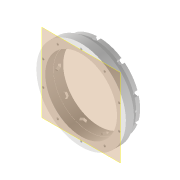
# Autodesk Inventor part: Anglerfish_3inch_tube_endpiece
Saved by Autodesk Inventor 2022 (Build 260153000, 153)
## iProperties
Created: 2022-04-12
Part Number: Anglerfish_3inch_tube_endpiece
Material: Generic
Document SubType Name: Modeling
Designer: Prakash Lab
Density: 1 g/cm^3
Appearance: Default
Author: Prakash Lab
Autodesk Inventor part; units mm, degrees
ref_plane "YZ Plane" through (0, 0, 0) normal (1, 0, 0) x (0, 1, 0)
ref_plane "XZ Plane" through (0, 0, 0) normal (0, 1, 0) x (-1, 0, 0)
ref_plane "XY Plane" through (0, 0, 0) normal (0, 0, 1) x (1, 0, 0)
ref_plane "Work Plane1" through (0, 0, -3) normal (0, 0, 1) x (0, -1, 0)
sketch "Sketch1" plane through (0, 0, -3) normal (0, 0, 1) x (0, -1, 0)
  circle A0 centre (0, 0) radius 44.3 projected
  circle A1 centre (0, 0) radius 44.6
  circle A2 centre (0, 0) radius 55.6
  point P0 (0, 0)
  dimension "d0" = 0.3
  dimension "d1" = 11
  constraints: 2 centre point
  measures "d0" radial gap between concentric circles of A0 A1
  measures "d1" radial gap between concentric circles of A1 A2
extrude "Extrusion1" add sketch "Sketch1" against normal blind 10 contours A2
sketch "Sketch2" plane through (0, 0, -13) normal (0, 0, -1) x (-1, 0, 0)
  circle A0 centre (0, 0) radius 44.3 projected
  circle A1 centre (0, 0) radius 51.3
  point P0 (0, 0)
  dimension "d4" = 7
  constraints: 1 centre point
  measures "d4" radial gap between concentric circles of A0 A1
extrude "Extrusion2" add sketch "Sketch2" along normal blind 12
sketch "Sketch3" plane through (0, 0, 0) normal (1, 0, 0) x (0, 1, 0)
  line L0 (-51.3, -25) -> (51.3, -25) projected
  line L1 (51.3, -13) -> (-51.3, -13) projected
  line L2 (-55.6, -13) -> (55.6, -13) projected
  line L3 (55.6, -3) -> (-55.6, -3) projected
  circle A0 centre (0, -19) radius 1.45
  point P0 (0, 0)
  dimension "d7" = 2.9
  dimension "d8" = 6
  constraints: 1 centre point
  measures "d7" diameter of A0
  measures "d8" distance from line of A0.centre L0
extrude "Extrusion3" cut sketch "Sketch3" along normal through all both and the other way through all
sketch "Sketch4" plane through (0, 0, 0) normal (1, 0, 0) x (0, 1, 0)
  line L0 (-1.9269, -22.2506) -> (-3.8033, -19.0006)
  line L1 (-3.8033, -19.0006) -> (-1.9269, -15.7506)
  line L2 (-1.9269, -15.7506) -> (1.8259, -15.7506)
  line L3 (1.8259, -15.7506) -> (3.7023, -19.0006)
  line L4 (3.7023, -19.0006) -> (1.8259, -22.2506)
  line L5 (1.8259, -22.2506) -> (-1.9269, -22.2506)
  line L6 (-55.6, -13) -> (55.6, -13) projected
  point P0 (0, 0)
  point P1 (-0.0505, -19.0006)
  dimension "d11" = 6.5
  constraints: 12 end point, 1 parallel, 14 other
  measures "d11" distance between parallel lines of L5 L2
extrude "Extrusion4" cut sketch "Sketch4" along normal mid plane 96
chamfer "Chamfer1" distance 4 distance2 7 1 edges at (51.3, 0, -13) measured on face at (51.8, 0, -13)
pattern_circular "Circular Pattern1" count 10 over 360 about axis through (0, 0, -13) along (0, 0, -1) of "Extrusion4"
sketch "Sketch5" plane through (0, 0, -3) normal (0, 0, 1) x (1, 0, 0)
  circle A0 centre (0, 0) radius 55.6 projected
  circle A1 centre (0, 0) radius 44.3 projected
  circle A2 centre (0, 0) radius 49.6 construction
  circle A3 centre (0, 49.6) radius 1.45
  point P0 (0, 0)
  dimension "d20" = 6
  dimension "d21" = 2.9
  constraints: 1 centre point, 1 vertical alignment, 2 other
  measures "d21" diameter of A3
extrude "Extrusion5" cut sketch "Sketch5" against normal blind 96 contours A3
sketch "Sketch6" plane through (0, 0, -25) normal (0, 0, -1) x (-1, 0, 0)
  circle A0 centre (0, 49.6) radius 1.45 projected
  line L0 (1.7321, 52.6) -> (3.4641, 49.6)
  line L1 (3.4641, 49.6) -> (1.7321, 46.6)
  line L2 (1.7321, 46.6) -> (-1.7321, 46.6)
  line L3 (-1.7321, 46.6) -> (-3.4641, 49.6)
  line L4 (-3.4641, 49.6) -> (-1.7321, 52.6)
  line L5 (-1.7321, 52.6) -> (1.7321, 52.6)
  line L6 (77.84, 0) -> (-77.84, 0) projected
  point P0 (0, 0)
  dimension "d27" = 6
  constraints: 12 end point, 1 coincident, 1 parallel, 13 other
  measures "d27" distance between parallel lines of L2 L5
extrude "Extrusion6" cut sketch "Sketch6" against normal blind 8
pattern_circular "Circular Pattern3" count 10 over 360 about axis through (0, 0, -3) along (0, 0, -1) of "Extrusion5", "Extrusion6"
body "Solid1"
